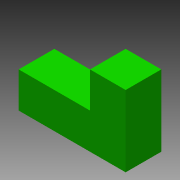
# Autodesk Inventor part: Part3
Saved by Autodesk Inventor 2013 (Build 170138000, 138)
## iProperties
Created: 2013-11-13
Part Number: Part3
Material: Generic
Document SubType Name: Modeling
Designer: s601298
Density: 1 g/cm^3
Mass: 27.6532 g
Surface Area: 65.3224 cm^2
Volume: 27.6532 cm^3
Author: s601298
Autodesk Inventor part; units mm, degrees
ref_plane "YZ Plane" through (0, 0, 0) normal (1, 0, 0) x (0, 1, 0)
ref_plane "XZ Plane" through (0, 0, 0) normal (0, 1, 0) x (-1, 0, 0)
ref_plane "XY Plane" through (0, 0, 0) normal (0, 0, 1) x (1, 0, 0)
sketch "Sketch1" plane through (0, 0, 0) normal (0, 1, 0) x (-1, 0, 0)
  line L0 (-10.4756, 4.2697) -> (46.6744, 4.2697)
  line L1 (46.6744, 4.2697) -> (46.6744, -14.7803)
  line L2 (46.6744, -14.7803) -> (-10.4756, -14.7803)
  line L3 (-10.4756, -14.7803) -> (-10.4756, 4.2697)
  point P0 (0, 0)
  dimension "d0" = 57.15
  dimension "d1" = 19.05
  constraints: 8 end point, 2 parallel, 1 horizontal, 1 perpendicular
  measures "d0" distance of L1.end L2.end
  measures "d1" distance of L0.end L1.end
extrude "Extrusion1" add sketch "Sketch1" along normal blind 19.05
sketch "Sketch2" plane through (0, 19.05, 0) normal (0, 1, 0) x (1, 0, 0)
  line L0 (10.4756, 14.7803) -> (-8.5744, 14.7803)
  line L1 (-8.5744, 14.7803) -> (-8.5744, -4.2697)
  line L2 (-8.5744, -4.2697) -> (10.4756, -4.2697)
  line L3 (10.4756, -4.2697) -> (10.4756, 14.7803)
  point P0 (0, 0)
  dimension "d4" = 19.05
  dimension "d5" = 19.05
  constraints: 8 end point, 2 parallel, 1 horizontal, 1 perpendicular
  measures "d4" distance of L2.end L1.end
  measures "d5" distance of L1.end L0.end
extrude "Extrusion2" add sketch "Sketch2" along normal blind 19.05
body "Solid1"
